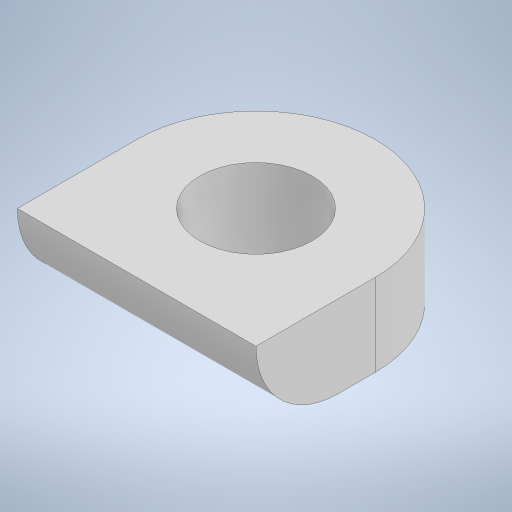
# Autodesk Inventor part: top_housing_screw_spacers
Saved by Autodesk Inventor 2023.1 (Build 271208000, 208)
## iProperties
Created: 2026-04-28
Part Number: top_housing_screw_spacers
Material: Generic
Document SubType Name: Modeling
Designer: Lars
Density: 1 g/cm^3
Appearance: Default
Author: Lars
Autodesk Inventor part; units mm, degrees
ref_plane "YZ Plane" through (0, 0, 0) normal (1, 0, 0) x (0, 1, 0)
ref_plane "XZ Plane" through (0, 0, 0) normal (0, 1, 0) x (-1, 0, 0)
ref_plane "XY Plane" through (0, 0, 0) normal (0, 0, 1) x (1, 0, 0)
sketch "Sketch1" plane through (0, 0, 0) normal (0, 1, 0) x (-1, 0, 0)
  circle A0 centre (0, 0) radius 2.05
  arc A1 (0, 4.35) -> (-4.35, 0) centre (0, 0) ccw construction
  line L0 (0, 4.35) -> (4.35, 4.35)
  line L1 (4.35, 0) -> (4.35, 4.35)
  line L2 (0, 4.35) -> (-4.35, 4.35)
  line L3 (-4.35, 0) -> (-4.35, 4.35)
  arc A2 (4.35, 0) -> (0, 4.35) centre (0, 0) ccw construction
  arc A3 (-4.35, 0) -> (4.35, 0) centre (0, 0) ccw
  dimension "d0" = 4.1
  dimension "d1" = 2.3
  constraints: 8 end point, 6 point on circle, 6 tangent, 4 centre point, 2 horizontal, 2 vertical, 1 coincident
  measures "d0" diameter of A0
  measures "d1" radial gap between concentric circles of A0 A1
extrude "Extrusion1" add sketch "Sketch1" along normal blind 3
fillet "Fillet1" radius 3 1 edges at (-2.175, 0, 4.35)
body "Solid1"
